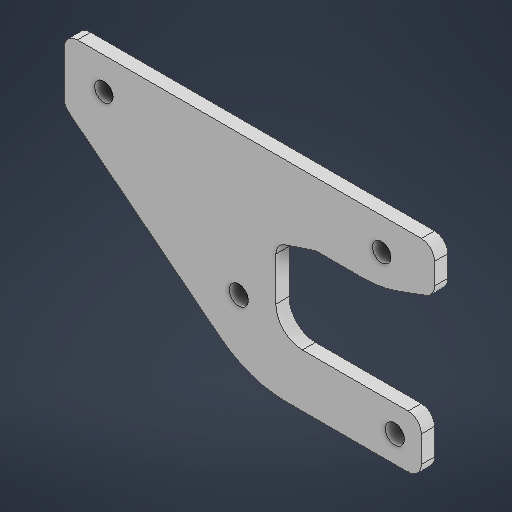
# Autodesk Inventor part: Goal Jaw Chassis
Saved by Autodesk Inventor 2025 (Build 290162000, 162)
## iProperties
Created: 2025-02-08
Part Number: Goal Jaw Chassis
Material: Generic
Document SubType Name: Modeling
Designer: Juan
Density: 1 g/cm^3
Appearance: Default
Author: Juan
Autodesk Inventor part; units mm, degrees
ref_plane "YZ Plane" through (0, 0, 0) normal (1, 0, 0) x (0, 1, 0)
ref_plane "XZ Plane" through (0, 0, 0) normal (0, 1, 0) x (-1, 0, 0)
ref_plane "XY Plane" through (0, 0, 0) normal (0, 0, 1) x (1, 0, 0)
sketch "Sketch1" plane through (0, 0, 0) normal (0, 0, 1) x (1, 0, 0)
  line L0 (0, 0) -> (-88.9, 0)
  line L1 (0, 0) -> (0, 15.24)
  line L2 (0, 15.24) -> (-88.9, 15.24)
  line L3 (-88.9, 15.24) -> (-88.9, 0)
  line L4 (0, 0) -> (-44.45, 0)
  line L5 (-44.45, 0) -> (-44.45, -22.225)
  line L6 (0, 0) -> (-31.75, 0)
  line L7 (-31.75, 0) -> (-31.75, -22.225)
  line L8 (-44.45, -22.225) -> (-31.75, -22.225)
  line L9 (-31.75, -22.225) -> (0, -22.225)
  line L10 (0, -22.225) -> (0, -34.925)
  line L11 (0, -34.925) -> (-44.45, -34.925)
  line L12 (-44.45, -34.925) -> (-88.9, 0)
  line L13 (0, -28.575) -> (-9.525, -28.575)
  circle A0 centre (-9.525, -28.575) radius 2.3241
  line L14 (-49.0828, -48.0247) -> (-25.6113, -57.7328)
  line L15 (-44.45, 0) -> (-38.1, 0)
  line L16 (-38.1, 0) -> (-38.1, -22.225)
  line L17 (0, -28.575) -> (-3.175, -28.575)
  line L18 (-3.175, -22.225) -> (-3.175, -34.925)
  dimension "d0" = 88.9
  dimension "d1" = 15.24
  dimension "d2" = 44.45
  dimension "d3" = 22.225
  dimension "d4" = 31.75
  dimension "d5" = 12.7
  dimension "d6" = 9.525
  dimension "d7" = 4.6482
  dimension "d8" = 25.4
  dimension "d13" = 3.175
  constraints: 38 end point, 5 point on line, 4 horizontal, 4 perpendicular, 3 midpoint, 3 vertical, 1 centre point, 1 coincident
  measures "d0" distance of L0.start L0.end
  measures "d1" distance of L0.start L1.end
  measures "d2" distance of L0.start L4.end
  measures "d3" distance of L4.end L5.end
  measures "d4" distance of L0.start L6.end
  measures "d5" distance of L9.end L10.end
  measures "d6" distance of L13.start L13.end
  measures "d7" diameter of A0
  measures "d8" distance of L14.start L14.end
  measures "d13" distance of L13.start L17.end
extrude "Extrusion1" add sketch "Sketch1" along normal blind 3.175
extrude "Extrusion2" cut sketch "Sketch1" along normal blind 3.175 contours L7 L8 L16 L0
extrude "Extrusion3" cut sketch "Sketch1" along normal blind 3.175 contours L9 L10 L13 L18 | L13 L10 L11 L18
fillet "Fillet1" radius 3.175 2 edges at (-3.175, -22.225, 1.5875) (-3.175, -34.925, 1.5875)
chamfer "Chamfer1" distance 3.175 distance2 9.525 1 edges at (-38.1, 0, 1.5875) measured on face at (-38.1, -7.4083, 2.1167)
fillet "Fillet2" radius 3.175 2 edges at (-38.1, -3.175, 1.5875) (-28.575, 0, 1.5875)
fillet "Fillet3" radius 6.35 1 edges at (-38.1, -22.225, 1.5875)
fillet "Fillet4" radius 25.4 1 edges at (-44.45, -34.925, 1.5875)
sketch "Sketch2" plane through (0, 0, 3.175) normal (0, 0, 1) x (1, 0, 0)
  circle A0 centre (-9.525, -28.575) radius 2.3241 projected
  arc A1 (-51.3577, -29.4975) -> (-35.6651, -34.925) centre (-35.6651, -9.525) ccw projected
  line L0 (-35.6651, -34.925) -> (-6.35, -34.925) projected
  arc A2 (-6.35, -34.925) -> (-3.175, -31.75) centre (-6.35, -31.75) ccw projected
  line L1 (-3.175, -31.75) -> (-3.175, -25.4) projected
  arc A3 (-3.175, -25.4) -> (-6.35, -22.225) centre (-6.35, -25.4) ccw projected
  line L2 (-6.35, -22.225) -> (-31.75, -22.225) projected
  arc A4 (-38.1, -15.875) -> (-31.75, -22.225) centre (-31.75, -15.875) ccw projected
  line L3 (-38.1, -15.875) -> (-38.1, -5.4634) projected
  arc A5 (-35.929, -2.4513) -> (-38.1, -5.4634) centre (-34.925, -5.4634) ccw projected
  line L4 (-29.0638, -0.1629) -> (-35.929, -2.4513) projected
  arc A6 (-28.0598, 0) -> (-29.0638, -0.1629) centre (-28.0598, -3.175) ccw projected
  line L5 (-28.0598, 0) -> (0, 0) projected
  line L6 (0, 0) -> (0, 15.24) projected
  line L7 (0, 15.24) -> (-88.9, 15.24) projected
  line L8 (-88.9, 15.24) -> (-88.9, 0) projected
  line L9 (-88.9, 0) -> (-51.3577, -29.4975) projected
  line L10 (0, 0) -> (0, 15.24) projected
  line L11 (0, 7.62) -> (-12.7, 7.62)
  circle A7 centre (-12.7, 7.62) radius 2.2225
  line L12 (-88.9, 7.62) -> (-79.375, 7.62)
  circle A8 centre (-79.375, 7.62) radius 2.2225
  dimension "d23" = 4.445
  dimension "d24" = 9.525
  dimension "d25" = 4.445
  dimension "d28" = 12.7
  constraints: 4 end point, 2 centre point, 2 coincident, 2 horizontal, 2 midpoint
  measures "d23" diameter of A7
  measures "d24" distance of L12.start L12.end
  measures "d25" diameter of A8
  measures "d28" distance of L11.start L11.end
extrude "Extrusion4" cut sketch "Sketch2" against normal blind 3.175 contours A7 | A8
chamfer "Chamfer2" distance 12.7 distance2 4.7625 1 edges at (0, 0, 1.5875) measured on face at (-18.7065, 0, 2.1167)
fillet "Fillet5" radius 25.4 1 edges at (-12.7, 0, 1.5875)
fillet "Fillet6" radius 3.175 1 edges at (0, 4.7625, 1.5875)
fillet "Fillet7" radius 3.175 1 edges at (0, 15.24, 1.5875)
fillet "Fillet8" radius 3.175 2 edges at (-88.9, 15.24, 1.5875) (-88.9, 0, 1.5875)
sketch "Sketch3" plane through (0, 0, 3.175) normal (0, 0, 1) x (1, 0, 0)
  arc A0 (-88.9, 1.5432) -> (-87.6866, -0.9534) centre (-85.725, 1.5432) ccw projected
  line L0 (-87.6866, -0.9534) -> (-51.3577, -29.4975) projected
  arc A1 (-51.3577, -29.4975) -> (-35.6651, -34.925) centre (-35.6651, -9.525) ccw projected
  line L1 (-35.6651, -34.925) -> (-6.35, -34.925) projected
  arc A2 (-6.35, -34.925) -> (-3.175, -31.75) centre (-6.35, -31.75) ccw projected
  line L2 (-3.175, -31.75) -> (-3.175, -25.4) projected
  arc A3 (-3.175, -25.4) -> (-6.35, -22.225) centre (-6.35, -25.4) ccw projected
  line L3 (-6.35, -22.225) -> (-31.75, -22.225) projected
  arc A4 (-38.1, -15.875) -> (-31.75, -22.225) centre (-31.75, -15.875) ccw projected
  line L4 (-38.1, -15.875) -> (-38.1, -5.4634) projected
  arc A5 (-35.929, -2.4513) -> (-38.1, -5.4634) centre (-34.925, -5.4634) ccw projected
  line L5 (-29.0638, -0.1629) -> (-35.929, -2.4513) projected
  arc A6 (-28.0598, 0) -> (-29.0638, -0.1629) centre (-28.0598, -3.175) ccw projected
  line L6 (-28.0598, 0) -> (-17.3059, 0) projected
  arc A7 (-17.3059, 0) -> (-8.3874, 1.6172) centre (-17.3059, 25.4) ccw projected
  line L7 (-2.0602, 3.9899) -> (-8.3874, 1.6172) projected
  arc A8 (-2.0602, 3.9899) -> (0, 6.9628) centre (-3.175, 6.9628) ccw projected
  line L8 (0, 6.9628) -> (0, 12.065) projected
  arc A9 (0, 12.065) -> (-3.175, 15.24) centre (-3.175, 12.065) ccw projected
  line L9 (-3.175, 15.24) -> (-85.725, 15.24) projected
  arc A10 (-85.725, 15.24) -> (-88.9, 12.065) centre (-85.725, 12.065) ccw projected
  line L10 (-88.9, 12.065) -> (-88.9, 1.5432) projected
  circle A11 centre (-12.7, 7.62) radius 2.2225 projected
  circle A12 centre (-79.375, 7.62) radius 2.2225 projected
  circle A13 centre (-9.525, -28.575) radius 2.3241 projected
  line L11 (-9.525, -28.575) -> (-46.99, -28.575)
  line L12 (-46.99, -28.575) -> (-46.99, -18.415)
  circle A14 centre (-46.99, -18.415) radius 2.3241
  point P0 (0, 0)
  dimension "d36" = 37.465
  dimension "d37" = 10.16
  dimension "d38" = 4.6482
  constraints: 4 end point, 1 centre point, 1 coincident, 1 horizontal, 1 perpendicular
  measures "d36" distance of L11.start L11.end
  measures "d37" distance of L11.end L12.end
  measures "d38" diameter of A14
extrude "Extrusion5" cut sketch "Sketch3" against normal blind 25.4 contours A14
body "Solid1"
